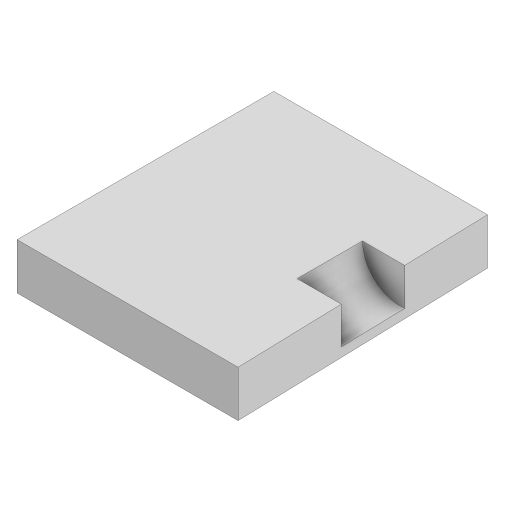
# Autodesk Inventor part: test_inventor_1
Saved by Autodesk Inventor 2024.3 (Build 283343000, 343)
## iProperties
Created: 2025-11-06
Part Number: test_inventor_1
Material: 常规
Document SubType Name: Modeling
Designer: lostcat
Density: 1 g/cm^3
Appearance: 默认
Author: lostcat
Autodesk Inventor part; units mm, degrees
ref_plane "YZ Plane" through (0, 0, 0) normal (1, 0, 0) x (0, 1, 0)
ref_plane "XZ Plane" through (0, 0, 0) normal (0, 1, 0) x (-1, 0, 0)
ref_plane "XY Plane" through (0, 0, 0) normal (0, 0, 1) x (1, 0, 0)
sketch "草图1" plane through (0, 0, 0) normal (0, 1, 0) x (-1, 0, 0)
  line L0 (-31.8679, 58.9557) -> (63.7358, 58.9557)
  line L1 (63.7358, 58.9557) -> (63.7358, -52.1268)
  line L2 (63.7358, -52.1268) -> (-28.6811, -52.1268)
  line L3 (-28.6811, -52.1268) -> (-31.8679, 58.9557)
  point P0 (0, 0)
  constraints: 8 end point, 2 perpendicular, 1 horizontal
extrude "拉伸1" add sketch "草图1" along normal blind 20
sketch "草图2" plane through (0, 20, 0) normal (0, 1, 0) x (1, 0, 0)
  line L0 (27.6987, -13.01) -> (11.4712, -13.01)
  line L1 (11.4712, -13.01) -> (11.4712, 15.2483)
  line L2 (11.4712, 15.2483) -> (27.6987, 15.2483)
  line L3 (27.6987, 15.2483) -> (27.6987, -13.01)
  point P0 (0, 0)
  constraints: 8 end point, 3 perpendicular, 1 horizontal
revolve "旋转1" cut sketch "草图2" angle 360 about axis through (27.6987, 20, -15.2483) along (0, 0, 1)
